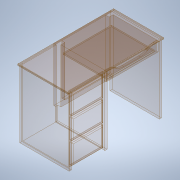
# Autodesk Inventor part: Work Table
Saved by Autodesk Inventor 2020 (Build 240168000, 168)
## iProperties
Created: 2021-01-02
Part Number: Work Table
Material: Generic
Document SubType Name: Modeling
Designer: frost
Density: 1 g/cm^3
Appearance: Polycarbonate - Smoked
Author: frost
Autodesk Inventor part; units mm, degrees
ref_plane "YZ Plane" through (0, 0, 0) normal (1, 0, 0) x (0, 1, 0)
sketch "Sketch1" plane through (0, 0, 0) normal (0, 1, 0) x (-1, 0, 0)
  line L0 (280, 535) -> (-280, 535)
  line L1 (-280, 535) -> (-280, -535)
  line L2 (-280, -535) -> (280, -535)
  line L3 (280, -535) -> (280, 535)
  line L4 (280, 535) -> (-280, -535) construction
  line L5 (-280, 535) -> (280, -535) construction
  point P0 (0, 0)
  dimension "d0" = 560
  dimension "d1" = 1070
  constraints: 12 end point, 2 midpoint, 2 parallel, 1 horizontal, 1 perpendicular
  measures "d0" distance of L2.end L1.end
  measures "d1" distance of L1.end L0.end
extrude "Extrusion1" add sketch "Sketch1" along normal blind 20
fillet "Fillet1" radius 5 12 edges at (280, 20, 0) (0, 20, -535) (280, 0, 0) (0, 20, 535) (-280, 20, 0) (-280, 0, 0) (0, 0, 535) (0, 0, -535) (280, 10, -535) (280, 10, 535) (-280, 10, -535) (-280, 10, 535)
sketch "Sketch2" plane through (0, 0, 0) normal (0, -1, 0) x (1, 0, 0)
  line L0 (275, 515) -> (-275, 515)
  line L1 (-275, 515) -> (-275, 490)
  line L2 (-275, 490) -> (275, 490)
  line L3 (275, 490) -> (275, 515)
  line L4 (-280, 530) -> (-280, -530) projected
  line L5 (280, -530) -> (280, 530) projected
  line L6 (275, 535) -> (-275, 535) projected
  point P0 (0, 0)
  dimension "d5" = 5
  dimension "d6" = 5
  dimension "d7" = 20
  dimension "d8" = 25
  constraints: 8 end point, 2 parallel, 1 horizontal, 1 perpendicular
  measures "d5" distance between parallel lines of L4 L1
  measures "d6" distance between parallel lines of L5 L3
  measures "d7" distance between parallel lines of L6 L0
  measures "d8" distance of L2.end L0.start
extrude "Extrusion2" add sketch "Sketch2" along normal blind 750
ref_plane "Work Plane1" through (-275, 5, 0) normal (0, 0, 1) x (1, 0, 0)
mirror "Mirror1" about plane through (-275, 5, 0) normal (0, 0, 1) of "Extrusion2"
ref_plane "Work Plane2" through (275, 0, 303) normal (0, 0, -1) x (-1, 0, 0)
mirror "Mirror2" about plane through (275, 0, 303) normal (0, 0, -1) of "Extrusion2"
sketch "Sketch3" plane through (-275, -750, 91) normal (-1, 0, 0) x (0, 0, 1)
  line L0 (-606, 750) -> (-621, 750) projected
  line L1 (25, 750) -> (25, 0) projected
  line L2 (-606, 750) -> (25, 750)
  line L3 (25, 750) -> (25, 150)
  line L4 (25, 150) -> (-606, 150)
  line L5 (-606, 150) -> (-606, 750)
  line L6 (-606, 0) -> (-581, 0) projected
  line L7 (-536, 750) -> (-45, 750)
  line L8 (-45, 750) -> (-45, 195)
  line L9 (-45, 195) -> (-536, 195)
  line L10 (-536, 195) -> (-536, 750)
  line L11 (-581, 750) -> (-581, 0) projected
  line L12 (0, 750) -> (0, 0) projected
  point P0 (-91, 750)
  point P1 (-581, 150)
  point P2 (0, 150)
  dimension "d12" = 150
  dimension "d13" = 45
  dimension "d14" = 45
  dimension "d15" = 45
  constraints: 16 end point, 4 parallel, 2 horizontal, 2 perpendicular, 2 point on line
  measures "d12" distance between parallel lines of L6 L4
  measures "d13" distance between parallel lines of L4 L9
  measures "d14" distance between parallel lines of L11 L10
  measures "d15" distance between parallel lines of L12 L8
extrude "Extrusion3" add sketch "Sketch3" along normal blind 20
extrude "Extrusion4" add sketch "Sketch3" against normal blind 35 contours L12 L4 L11 L2 L10 L9 L8
sketch "Sketch4" plane through (-240, -750, 91) normal (1, 0, 0) x (0, 0, -1)
  line L0 (25, 660) -> (559.852, 660)
  line L1 (584.852, 660) -> (584.852, 645)
  line L2 (559.852, 645) -> (25, 645)
  line L3 (25, 645) -> (25, 660)
  line L4 (0, 750) -> (581, 750) projected
  line L5 (559.852, 660) -> (559.852, 645)
  line L6 (0, 750) -> (0, 0) projected
  point P0 (91, 750)
  dimension "d20" = 90
  dimension "d21" = 15
  dimension "d22" = 25
  dimension "d23" = 25
  constraints: 10 end point, 2 parallel, 1 horizontal, 1 perpendicular, 1 vertical
  measures "d20" distance between parallel lines of L4 L0
  measures "d21" distance of L2.end L0.start
  measures "d22" distance between parallel lines of L1 L5
  measures "d23" distance between parallel lines of L6 L3
extrude "Extrusion5" add sketch "Sketch4" along normal blind 480
sketch "Sketch5" plane through (240, -750, 91) normal (1, 0, 0) x (0, 0, -1)
  line L0 (0, 150) -> (0, 750) projected
  line L1 (581, 750) -> (581, 150) projected
  line L2 (0, 642.2608) -> (581, 642.2608)
  line L3 (581, 642.2608) -> (581, 742.2608)
  line L4 (0, 742.2608) -> (0, 642.2608)
  line L5 (581, 742.2608) -> (549.0698, 742.2608)
  line L6 (581, 692.2608) -> (581, 742.2608)
  line L7 (0, 742.2608) -> (31.9302, 742.2608)
  line L8 (0, 692.2608) -> (0, 742.2608)
  line L9 (501, 742.2608) -> (501, 692.2608)
  line L10 (119.116, 714.3208) -> (110.884, 720.2008)
  line L11 (461.884, 714.3208) -> (470.116, 720.2008)
  line L12 (581, 742.2608) -> (549.0698, 742.2608)
  line L13 (31.9302, 742.2608) -> (0, 742.2608)
  line L14 (198.0698, 692.2608) -> (382.9302, 692.2608)
  arc A0 (119.116, 714.3208) -> (31.9302, 742.2608) centre (31.9302, 592.2608) ccw
  arc A1 (110.884, 720.2008) -> (198.0698, 692.2608) centre (198.0698, 842.2608) ccw
  arc A2 (382.9302, 692.2608) -> (470.116, 720.2008) centre (382.9302, 842.2608) ccw
  arc A3 (549.0698, 742.2608) -> (461.884, 714.3208) centre (549.0698, 592.2608) ccw
  point P0 (91, 750)
  point P1 (80, 742.2608)
  point P2 (0, 742.2608)
  dimension "d32" = 80
  dimension "d33" = 150
  constraints: 26 end point, 8 point on circle, 8 tangent, 7 point on line, 4 centre point, 4 horizontal, 3 equal radius, 3 parallel, 1 perpendicular
  measures "d32" distance between parallel lines of L6 L9
  measures "d33" radius of A0
extrude "Extrusion6" add sketch "Sketch5" along normal blind 22
sketch "Sketch6" plane through (275, -750, 116) normal (1, 0, 0) x (0, 0, -1)
  line L0 (-374, 750) -> (-374, 0) projected
  line L1 (0, 150) -> (0, 0) projected
  line L2 (-374, 750) -> (0, 750)
  line L3 (0, 750) -> (0, 9.717)
  line L4 (0, 9.717) -> (-374, 9.717)
  line L5 (-374, 9.717) -> (-374, 750)
  line L6 (-362, 730) -> (-12, 730)
  line L7 (-12, 730) -> (-12, 509.9057)
  line L8 (-12, 509.9057) -> (-362, 509.9057)
  line L9 (-362, 509.9057) -> (-362, 730)
  line L10 (-362, 489.9057) -> (-12, 489.9057)
  line L11 (-12, 489.9057) -> (-12, 269.8113)
  line L12 (-12, 269.8113) -> (-362, 269.8113)
  line L13 (-362, 269.8113) -> (-362, 489.9057)
  line L14 (-362, 249.8113) -> (-12, 249.8113)
  line L15 (-12, 249.8113) -> (-12, 29.717)
  line L16 (-12, 29.717) -> (-362, 29.717)
  line L17 (-362, 29.717) -> (-362, 249.8113)
  point P0 (116, 750)
  point P1 (-374, 9.717)
  dimension "d36" = 350
  dimension "d37" = 350
  dimension "d38" = 20
  dimension "d39" = 20
  dimension "d40" = 20
  dimension "d41" = 20
  dimension "d42" = 12
  dimension "d43" = 12
  dimension "d44" = 12
  dimension "d45" = 12
  constraints: 32 end point, 8 parallel, 4 horizontal, 4 perpendicular, 3 equal length, 3 point on line
  measures "d36" distance of L10.start L10.end
  measures "d37" distance of L7.end L8.end
  measures "d38" distance between parallel lines of L2 L6
  measures "d39" distance between parallel lines of L8 L10
  measures "d40" distance between parallel lines of L12 L14
  measures "d41" distance between parallel lines of L4 L16
  measures "d42" distance between parallel lines of L0 L17
  measures "d43" distance between parallel lines of L1 L15
  measures "d44" distance between parallel lines of L3 L7
  measures "d45" distance between parallel lines of L0 L9
extrude "Extrusion7" add sketch "Sketch6" against normal blind 540 contours L2 L3 L1 L4 L0 | L6 L7 L8 L9 | L10 L11 L12 L13 | L14 L15 L16 L17
extrude "Extrusion8" cut sketch "Sketch6" against normal blind 30
chamfer "Chamfer1" distance 10 angle 45 12 edges at (275, -240.0943, 303) (275, -130.0472, 478) (275, -20, 303) (275, -130.0472, 128) (275, -260.0943, 303) (275, -370.1415, 128) (275, -480.1887, 303) (275, -370.1415, 478) (275, -500.1887, 303) (275, -610.2359, 478) (275, -720.283, 303) (275, -610.2359, 128)
body "Solid1"
